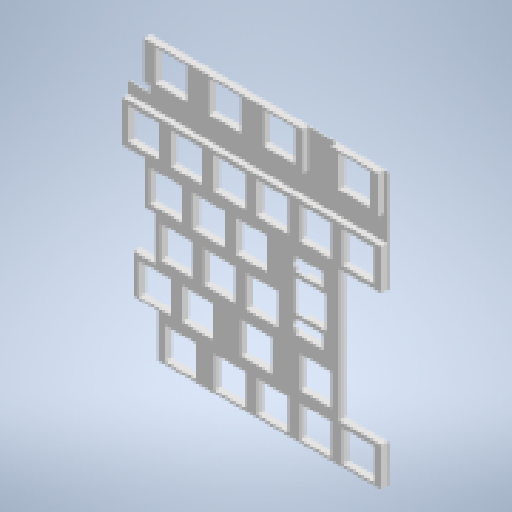
# Autodesk Inventor part: Right plate
Saved by Autodesk Inventor 2025 (Build 290162000, 162)
## iProperties
Created: 2024-08-01
Part Number: Right plate
Material: Generic
Document SubType Name: Modeling
Designer: adam
Density: 1 g/cm^3
Appearance: Default
Author: adam
Autodesk Inventor part; units mm, degrees
(part 1 of 2)
ref_plane "YZ Plane" through (0, 0, 0) normal (1, 0, 0) x (0, 1, 0)
ref_plane "XZ Plane" through (0, 0, 0) normal (0, 1, 0) x (-1, 0, 0)
ref_plane "XY Plane" through (0, 0, 0) normal (0, 0, 1) x (1, 0, 0)
sketch "Sketch1" plane through (0, 0, 0) normal (0, 0, 1) x (1, 0, 0)
  line L0 (210, -24.2525) -> (210, -19.005) construction
  line L1 (200.5, -24.2525) -> (210, -24.2525) construction
  line L2 (200.5, -29.5) -> (200.5, -24.2525) construction
  line L3 (200.5, -48.0525) -> (200.5, -29.5) construction
  line L4 (210.25, -48.0525) -> (200.5, -48.0525) construction
  line L5 (210.25, -67.1525) -> (210.25, -48.0525) construction
  line L6 (215, -67.1525) -> (210.25, -67.1525) construction
  line L7 (215, -86.2525) -> (215, -67.1525) construction
  line L8 (205.25, -86.2525) -> (215, -86.2525) construction
  line L9 (205.25, -103.805) -> (205.25, -86.2525) construction
  line L10 (216.3009, -103.805) -> (205.25, -103.805) construction
  line L11 (216.3009, -120.0025) -> (216.3009, -103.805) construction
  line L12 (210.1, -2) -> (210.1, -24.3525)
  line L13 (210.1, -24.3525) -> (200.6, -24.3525)
  line L14 (200.6, -24.3525) -> (200.6, -29.5)
  line L15 (200.6, -29.5) -> (200.6, -47.9525)
  line L16 (200.6, -47.9525) -> (210.35, -47.9525)
  line L17 (210.35, -47.9525) -> (210.35, -67.0525)
  line L18 (210.35, -67.0525) -> (215.1, -67.0525)
  line L19 (215.1, -67.0525) -> (215.1, -86.3525)
  line L20 (215.1, -86.3525) -> (205.35, -86.3525)
  line L21 (205.35, -86.3525) -> (205.35, -103.705)
  line L22 (205.35, -103.705) -> (216.4009, -103.705)
  line L23 (216.4009, -103.705) -> (216.4009, -123)
  line L24 (316, -2) -> (316, -123) projected
  line L25 (316, -2) -> (210.1, -2)
  line L26 (316, -123) -> (216.4009, -123)
  line L27 (316, -123) -> (0, -123) construction
  line L28 (316, -2) -> (316, -123) construction
  line L29 (0, -2) -> (316, -2) construction
  line L30 (0, -123) -> (0, -2) construction
  circle A0 centre (18.6, -119.6) radius 0.725 construction
  circle A1 centre (23, -114.9) radius 2.55 construction
  circle A2 centre (25.6, -120.65) radius 0.725 construction
  circle A3 centre (43.1, -119.6) radius 0.725 construction
  circle A4 centre (50.1, -120.65) radius 0.725 construction
  circle A5 centre (47.5, -114.9) radius 2.55 construction
  line L31 (67.3517, -120.975) -> (73.3517, -120.975) construction
  line L32 (67.3517, -105.975) -> (67.3517, -120.975) construction
  line L33 (73.3517, -105.975) -> (67.3517, -105.975) construction
  line L34 (73.3517, -120.975) -> (73.3517, -105.975) construction
  circle A6 centre (13.1, -100.5) radius 0.725 construction
  circle A7 centre (20.1, -101.55) radius 0.725 construction
  circle A8 centre (39.35, -100.5) radius 0.725 construction
  circle A9 centre (17.5, -95.8) radius 2.55 construction
  circle A10 centre (46.35, -101.55) radius 0.725 construction
  circle A11 centre (58.35, -100.5) radius 0.725 construction
  circle A12 centre (65.35, -101.55) radius 0.725 construction
  circle A13 centre (77.35, -100.5) radius 0.725 construction
  circle A14 centre (43.75, -95.8) radius 2.55 construction
  circle A15 centre (62.75, -95.8) radius 2.55 construction
  circle A16 centre (81.75, -95.8) radius 2.55 construction
  circle A17 centre (132.4518, -119.675) radius 0.725 construction
  circle A18 centre (139.4518, -120.725) radius 0.725 construction
  circle A19 centre (136.8518, -114.975) radius 2.55 construction
  circle A20 centre (84.35, -101.55) radius 0.725 construction
  circle A21 centre (96.35, -100.5) radius 0.725 construction
  circle A22 centre (103.35, -101.55) radius 0.725 construction
  circle A23 centre (115.35, -100.5) radius 0.725 construction
  circle A24 centre (100.75, -95.8) radius 2.55 construction
  circle A25 centre (119.75, -95.8) radius 2.55 construction
  circle A26 centre (122.35, -101.55) radius 0.725 construction
  circle A27 centre (134.35, -100.5) radius 0.725 construction
  circle A28 centre (141.35, -101.55) radius 0.725 construction
  circle A29 centre (153.35, -100.5) radius 0.725 construction
  circle A30 centre (138.75, -95.8) radius 2.55 construction
  circle A31 centre (157.75, -95.8) radius 2.55 construction
  circle A32 centre (15.6, -82.45) radius 0.725 construction
  circle A33 centre (8.6, -81.4) radius 0.725 construction
  circle A34 centre (37.1, -82.45) radius 0.725 construction
  circle A35 centre (30.1, -81.4) radius 0.725 construction
  circle A36 centre (56.1, -82.45) radius 0.725 construction
  circle A37 centre (49.1, -81.4) radius 0.725 construction
  circle A38 centre (75.1, -82.45) radius 0.725 construction
  circle A39 centre (68.1, -81.4) radius 0.725 construction
  circle A40 centre (13, -76.7) radius 2.55 construction
  circle A41 centre (34.5, -76.7) radius 2.55 construction
  circle A42 centre (53.5, -76.7) radius 2.55 construction
  circle A43 centre (72.5, -76.7) radius 2.55 construction
  circle A44 centre (94.1, -82.45) radius 0.725 construction
  circle A45 centre (87.1, -81.4) radius 0.725 construction
  circle A46 centre (113.1, -82.45) radius 0.725 construction
  circle A47 centre (106.1, -81.4) radius 0.725 construction
  circle A48 centre (132.1, -82.45) radius 0.725 construction
  circle A49 centre (125.1, -81.4) radius 0.725 construction
  circle A50 centre (151.1, -82.45) radius 0.725 construction
  circle A51 centre (144.1, -81.4) radius 0.725 construction
  circle A52 centre (91.5, -76.7) radius 2.55 construction
  circle A53 centre (110.5, -76.7) radius 2.55 construction
  circle A54 centre (129.5, -76.7) radius 2.55 construction
  circle A55 centre (148.5, -76.7) radius 2.55 construction
  circle A56 centre (221.85, -119.6) radius 0.725 construction
  circle A57 centre (228.85, -120.65) radius 0.725 construction
  circle A58 centre (226.25, -114.9) radius 2.55 construction
  line L35 (200.3518, -120.975) -> (206.3518, -120.975) construction
  line L36 (200.3518, -105.975) -> (200.3518, -120.975) construction
  line L37 (206.3518, -105.975) -> (200.3518, -105.975) construction
  line L38 (206.3518, -120.975) -> (206.3518, -105.975) construction
  circle A59 centre (160.35, -101.55) radius 0.725 construction
  circle A60 centre (172.35, -100.5) radius 0.725 construction
  circle A61 centre (179.35, -101.55) radius 0.725 construction
  circle A62 centre (191.35, -100.5) radius 0.725 construction
  circle A63 centre (198.35, -101.55) radius 0.725 construction
  circle A64 centre (176.75, -95.8) radius 2.55 construction
  circle A65 centre (195.75, -95.8) radius 2.55 construction
  circle A66 centre (210.35, -100.5) radius 0.725 construction
  circle A67 centre (217.35, -101.55) radius 0.725 construction
  circle A68 centre (229.35, -100.5) radius 0.725 construction
  circle A69 centre (236.35, -101.55) radius 0.725 construction
  circle A70 centre (214.75, -95.8) radius 2.55 construction
  circle A71 centre (233.75, -95.8) radius 2.55 construction
  circle A72 centre (243.85, -119.6) radius 0.725 construction
  circle A73 centre (250.85, -120.65) radius 0.725 construction
  circle A74 centre (248.25, -114.9) radius 2.55 construction
  circle A75 centre (262.85, -119.6) radius 0.725 construction
  circle A76 centre (269.85, -120.65) radius 0.725 construction
  circle A77 centre (267.25, -114.9) radius 2.55 construction
  circle A78 centre (281.85, -119.6) radius 0.725 construction
  circle A79 centre (288.85, -120.65) radius 0.725 construction
  circle A80 centre (286.25, -114.9) radius 2.55 construction
  circle A81 centre (300.85, -119.6) radius 0.725 construction
  circle A82 centre (307.85, -120.65) radius 0.725 construction
  circle A83 centre (305.25, -114.9) radius 2.55 construction
  circle A84 centre (255.6, -100.5) radius 0.725 construction
  circle A85 centre (262.6, -101.55) radius 0.725 construction
  circle A86 centre (260, -95.8) radius 2.55 construction
  circle A87 centre (281.85, -100.5) radius 0.725 construction
  circle A88 centre (288.85, -101.55) radius 0.725 construction
  circle A89 centre (314, -102.5) radius 0.5 construction
  circle A90 centre (286.25, -95.8) radius 2.55 construction
  circle A91 centre (314, -99.96) radius 0.5 construction
  circle A92 centre (314, -97.42) radius 0.5 construction
  circle A93 centre (314, -94.88) radius 0.5 construction
  circle A94 centre (170.1, -82.45) radius 0.725 construction
  circle A95 centre (163.1, -81.4) radius 0.725 construction
  circle A96 centre (189.1, -82.45) radius 0.725 construction
  circle A97 centre (182.1, -81.4) radius 0.725 construction
  circle A98 centre (208.1, -82.45) radius 0.725 construction
  circle A99 centre (201.1, -81.4) radius 0.725 construction
  circle A100 centre (227.1, -82.45) radius 0.725 construction
  circle A101 centre (220.1, -81.4) radius 0.725 construction
  circle A102 centre (167.5, -76.7) radius 2.55 construction
  circle A103 centre (186.5, -76.7) radius 2.55 construction
  circle A104 centre (205.5, -76.7) radius 2.55 construction
  circle A105 centre (224.5, -76.7) radius 2.55 construction
  circle A106 centre (246.1, -82.45) radius 0.725 construction
  circle A107 centre (239.1, -81.4) radius 0.725 construction
  circle A108 centre (265.1, -82.45) radius 0.725 construction
  circle A109 centre (258.1, -81.4) radius 0.725 construction
  circle A110 centre (314, -92.34) radius 0.5 construction
  circle A111 centre (314, -89.8) radius 0.5 construction
  line L39 (275, -82.25) -> (290, -82.25) construction
  line L40 (275, -76.25) -> (275, -82.25) construction
  line L41 (290, -76.25) -> (275, -76.25) construction
  line L42 (290, -82.25) -> (290, -76.25) construction
  circle A112 centre (243.5, -76.7) radius 2.55 construction
  circle A113 centre (262.5, -76.7) radius 2.55 construction
  circle A114 centre (288.675, -71.675) radius 0.725 construction
  circle A115 centre (283.975, -67.275) radius 2.55 construction
  circle A116 centre (289.725, -64.675) radius 0.725 construction
  circle A117 centre (22.6, -63.35) radius 0.725 construction
  circle A118 centre (15.6, -62.3) radius 0.725 construction
  circle A119 centre (20, -57.6) radius 2.55 construction
  line L43 (5, -63.6) -> (11, -63.6) construction
  line L44 (5, -48.6) -> (5, -63.6) construction
  line L45 (11, -48.6) -> (5, -48.6) construction
  line L46 (11, -63.6) -> (11, -48.6) construction
  line L47 (29, -63.6) -> (35, -63.6) construction
  line L48 (29, -48.6) -> (29, -63.6) construction
  line L49 (35, -48.6) -> (29, -48.6) construction
  line L50 (35, -63.6) -> (35, -48.6) construction
  circle A120 centre (51.35, -63.35) radius 0.725 construction
  circle A121 centre (44.35, -62.3) radius 0.725 construction
  circle A122 centre (48.75, -57.6) radius 2.55 construction
  circle A123 centre (70.35, -63.35) radius 0.725 construction
  circle A124 centre (63.35, -62.3) radius 0.725 construction
  circle A125 centre (82.35, -62.3) radius 0.725 construction
  circle A126 centre (67.75, -57.6) radius 2.55 construction
  circle A127 centre (10.6, -43.2) radius 0.725 construction
  circle A128 centre (17.6, -44.25) radius 0.725 construction
  circle A129 centre (34.6, -43.2) radius 0.725 construction
  circle A130 centre (41.6, -44.25) radius 0.725 construction
  circle A131 centre (15, -38.5) radius 2.55 construction
  circle A132 centre (39, -38.5) radius 2.55 construction
  circle A133 centre (53.6, -43.2) radius 0.725 construction
  circle A134 centre (60.6, -44.25) radius 0.725 construction
  circle A135 centre (72.6, -43.2) radius 0.725 construction
  circle A136 centre (79.6, -44.25) radius 0.725 construction
  circle A137 centre (58, -38.5) radius 2.55 construction
  circle A138 centre (77, -38.5) radius 2.55 construction
  circle A139 centre (89.35, -63.35) radius 0.725 construction
  circle A140 centre (101.35, -62.3) radius 0.725 construction
  circle A141 centre (86.75, -57.6) radius 2.55 construction
  circle A142 centre (108.35, -63.35) radius 0.725 construction
  circle A143 centre (120.35, -62.3) radius 0.725 construction
  circle A144 centre (105.75, -57.6) radius 2.55 construction
  circle A145 centre (127.35, -63.35) radius 0.725 construction
  circle A146 centre (139.35, -62.3) radius 0.725 construction
  circle A147 centre (124.75, -57.6) radius 2.55 construction
  circle A148 centre (146.35, -63.35) radius 0.725 construction
  circle A149 centre (158.35, -62.3) radius 0.725 construction
  circle A150 centre (143.75, -57.6) radius 2.55 construction
  circle A151 centre (91.6, -43.2) radius 0.725 construction
  circle A152 centre (98.6, -44.25) radius 0.725 construction
  circle A153 centre (110.6, -43.2) radius 0.725 construction
  circle A154 centre (117.6, -44.25) radius 0.725 construction
  circle A155 centre (96, -38.5) radius 2.55 construction
  circle A156 centre (115, -38.5) radius 2.55 construction
  circle A157 centre (129.6, -43.2) radius 0.725 construction
  circle A158 centre (136.6, -44.25) radius 0.725 construction
  circle A159 centre (148.6, -43.2) radius 0.725 construction
  circle A160 centre (155.6, -44.25) radius 0.725 construction
  circle A161 centre (134, -38.5) radius 2.55 construction
  circle A162 centre (153, -38.5) radius 2.55 construction
  circle A163 centre (8.1, -14.7) radius 0.725 construction
  circle A164 centre (15.1, -15.75) radius 0.725 construction
  circle A165 centre (41.1, -14.7) radius 0.725 construction
  circle A166 centre (12.5, -10) radius 2.55 construction
  circle A167 centre (48.1, -15.75) radius 0.725 construction
  circle A168 centre (65.1, -14.7) radius 0.725 construction
  circle A169 centre (72.1, -15.75) radius 0.725 construction
  circle A170 centre (45.5, -10) radius 2.55 construction
  circle A171 centre (69.5, -10) radius 2.55 construction
  circle A172 centre (123.5, -26.25) radius 0.425 construction
  circle A173 centre (126, -26.25) radius 0.425 construction
  circle A174 centre (128.5, -26.25) radius 0.425 construction
  circle A175 centre (131, -26.25) radius 0.425 construction
  circle A176 centre (133.5, -26.25) radius 0.425 construction
  circle A177 centre (136, -26.25) radius 0.425 construction
  circle A178 centre (138.5, -26.25) radius 0.425 construction
  circle A179 centre (122.25, -23.75) radius 0.425 construction
  circle A180 centre (124.75, -23.75) radius 0.425 construction
  circle A181 centre (127.25, -23.75) radius 0.425 construction
  circle A182 centre (129.75, -23.75) radius 0.425 construction
  circle A183 centre (132.25, -23.75) radius 0.425 construction
  circle A184 centre (134.75, -23.75) radius 0.425 construction
  circle A185 centre (137.25, -23.75) radius 0.425 construction
  circle A186 centre (139.75, -23.75) radius 0.425 construction
  circle A187 centre (141, -26.25) radius 0.425 construction
  circle A188 centre (143.5, -26.25) radius 0.425 construction
  circle A189 centre (146, -26.25) radius 0.425 construction
  circle A190 centre (148.5, -26.25) radius 0.425 construction
  circle A191 centre (151, -26.25) radius 0.425 construction
  circle A192 centre (153.5, -26.25) radius 0.425 construction
  circle A193 centre (156, -26.25) radius 0.425 construction
  circle A194 centre (158.5, -26.25) radius 0.425 construction
  circle A195 centre (142.25, -23.75) radius 0.425 construction
  circle A196 centre (144.75, -23.75) radius 0.425 construction
  circle A197 centre (147.25, -23.75) radius 0.425 construction
  circle A198 centre (149.75, -23.75) radius 0.425 construction
  circle A199 centre (152.25, -23.75) radius 0.425 construction
  circle A200 centre (154.75, -23.75) radius 0.425 construction
  circle A201 centre (157.25, -23.75) radius 0.425 construction
  circle A202 centre (89.1, -14.7) radius 0.725 construction
  circle A203 centre (96.1, -15.75) radius 0.725 construction
  circle A204 centre (113.1, -14.7) radius 0.725 construction
  circle A205 centre (120.1, -15.75) radius 0.725 construction
  circle A206 centre (93.5, -10) radius 2.55 construction
  circle A207 centre (117.5, -10) radius 2.55 construction
  circle A208 centre (137.1, -14.7) radius 0.725 construction
  circle A209 centre (144.1, -15.75) radius 0.725 construction
  circle A210 centre (141.5, -10) radius 2.55 construction
  circle A211 centre (165.35, -63.35) radius 0.725 construction
  circle A212 centre (177.35, -62.3) radius 0.725 construction
  circle A213 centre (162.75, -57.6) radius 2.55 construction
  circle A214 centre (184.35, -63.35) radius 0.725 construction
  circle A215 centre (196.35, -62.3) radius 0.725 construction
  circle A216 centre (181.75, -57.6) radius 2.55 construction
  circle A217 centre (203.35, -63.35) radius 0.725 construction
  circle A218 centre (215.35, -62.3) radius 0.725 construction
  circle A219 centre (200.75, -57.6) radius 2.55 construction
  circle A220 centre (222.35, -63.35) radius 0.725 construction
  circle A221 centre (234.35, -62.45) radius 0.725 construction
  circle A222 centre (219.75, -57.6) radius 2.55 construction
  circle A223 centre (167.6, -43.2) radius 0.725 construction
  circle A224 centre (174.6, -44.25) radius 0.725 construction
  circle A225 centre (186.6, -43.2) radius 0.725 construction
  circle A226 centre (193.6, -44.25) radius 0.725 construction
  circle A227 centre (172, -38.5) radius 2.55 construction
  circle A228 centre (191, -38.5) radius 2.55 construction
  circle A229 centre (205.6, -43.2) radius 0.725 construction
  circle A230 centre (212.6, -44.25) radius 0.725 construction
  circle A231 centre (224.6, -43.2) radius 0.725 construction
  circle A232 centre (231.6, -44.25) radius 0.725 construction
  circle A233 centre (210, -38.5) radius 2.55 construction
  circle A234 centre (229, -38.5) radius 2.55 construction
  circle A235 centre (241.35, -63.5) radius 0.725 construction
  circle A236 centre (253.35, -62.4466) radius 0.725 construction
  circle A237 centre (238.75, -57.75) radius 2.55 construction
  circle A238 centre (260.35, -63.4966) radius 0.725 construction
  circle A239 centre (257.75, -57.7466) radius 2.55 construction
  line L51 (275, -58.25) -> (290, -58.25) construction
  line L52 (275, -52.25) -> (275, -58.25) construction
  line L53 (290, -52.25) -> (275, -52.25) construction
  line L54 (290, -58.25) -> (290, -52.25) construction
  circle A240 centre (243.6, -43.2) radius 0.725 construction
  circle A241 centre (250.6, -44.25) radius 0.725 construction
  circle A242 centre (262.6, -43.2) radius 0.725 construction
  circle A243 centre (269.6, -44.25) radius 0.725 construction
  circle A244 centre (248, -38.5) radius 2.55 construction
  circle A245 centre (267, -38.5) radius 2.55 construction
  circle A246 centre (281.6, -43.2) radius 0.725 construction
  circle A247 centre (288.6, -44.25) radius 0.725 construction
  circle A248 centre (300.6, -43.2) radius 0.725 construction
  circle A249 centre (307.6, -44.25) radius 0.725 construction
  circle A250 centre (286, -38.5) radius 2.55 construction
  circle A251 centre (305, -38.5) radius 2.55 construction
  circle A252 centre (161, -26.25) radius 0.425 construction
  circle A253 centre (159.75, -23.75) radius 0.425 construction
  circle A254 centre (219, -34) radius 1.6 construction
  circle A255 centre (169.6, -14.7) radius 0.725 construction
  circle A256 centre (176.6, -15.75) radius 0.725 construction
  circle A257 centre (193.6, -14.7) radius 0.725 construction
  circle A258 centre (174, -10) radius 2.55 construction
  circle A259 centre (198, -10) radius 2.55 construction
  circle A260 centre (200.6, -15.75) radius 0.725 construction
  circle A261 centre (217.6, -14.7) radius 0.725 construction
  circle A262 centre (224.6, -15.75) radius 0.725 construction
  circle A263 centre (222, -10) radius 2.55 construction
  circle A264 centre (241.6, -14.7) radius 0.725 construction
  circle A265 centre (248.6, -15.75) radius 0.725 construction
  circle A266 centre (265.6, -14.7) radius 0.725 construction
  circle A267 centre (272.6, -15.75) radius 0.725 construction
  circle A268 centre (246, -10) radius 2.55 construction
  circle A269 centre (270, -10) radius 2.55 construction
  circle A270 centre (299.1, -14.7) radius 0.725 construction
  circle A271 centre (306.1, -15.75) radius 0.725 construction
  circle A272 centre (303.5, -10) radius 2.55 construction
  line L55 (214.9975, -2.9975) -> (229.0025, -2.9975)
  line L56 (229.0025, -2.9975) -> (229.0025, -17.0025)
  line L57 (229.0025, -17.0025) -> (214.9975, -17.0025)
  line L58 (214.9975, -17.0025) -> (214.9975, -2.9975)
  line L59 (214.9975, -2.9975) -> (229.0025, -17.0025) construction
  line L60 (229.0025, -2.9975) -> (214.9975, -17.0025) construction
  line L61 (238.9975, -2.9975) -> (253.0025, -2.9975)
  line L62 (253.0025, -2.9975) -> (253.0025, -17.0025)
  line L63 (253.0025, -17.0025) -> (238.9975, -17.0025)
  line L64 (238.9975, -17.0025) -> (238.9975, -2.9975)
  line L65 (238.9975, -2.9975) -> (253.0025, -17.0025) construction
  line L66 (253.0025, -2.9975) -> (238.9975, -17.0025) construction
  line L67 (262.9975, -2.9975) -> (277.0025, -2.9975)
  line L68 (277.0025, -2.9975) -> (277.0025, -17.0025)
  line L69 (277.0025, -17.0025) -> (262.9975, -17.0025)
  line L70 (262.9975, -17.0025) -> (262.9975, -2.9975)
  line L71 (262.9975, -2.9975) -> (277.0025, -17.0025) construction
  line L72 (277.0025, -2.9975) -> (262.9975, -17.0025) construction
  line L73 (296.4975, -2.9975) -> (310.5025, -2.9975)
  line L74 (310.5025, -2.9975) -> (310.5025, -17.0025)
  line L75 (310.5025, -17.0025) -> (296.4975, -17.0025)
  line L76 (296.4975, -17.0025) -> (296.4975, -2.9975)
  line L77 (296.4975, -2.9975) -> (310.5025, -17.0025) construction
  line L78 (310.5025, -2.9975) -> (296.4975, -17.0025) construction
  line L79 (202.9975, -31.4975) -> (217.0025, -31.4975)
  line L80 (217.0025, -31.4975) -> (217.0025, -45.5025)
  line L81 (217.0025, -45.5025) -> (202.9975, -45.5025)
  line L82 (202.9975, -45.5025) -> (202.9975, -31.4975)
  line L83 (202.9975, -31.4975) -> (217.0025, -45.5025) construction
  line L84 (217.0025, -31.4975) -> (202.9975, -45.5025) construction
  line L85 (221.9975, -31.4975) -> (236.0025, -31.4975)
  line L86 (236.0025, -31.4975) -> (236.0025, -45.5025)
  line L87 (236.0025, -45.5025) -> (221.9975, -45.5025)
  line L88 (221.9975, -45.5025) -> (221.9975, -31.4975)
  line L89 (221.9975, -31.4975) -> (236.0025, -45.5025) construction
  line L90 (236.0025, -31.4975) -> (221.9975, -45.5025) construction
  line L91 (240.9975, -31.4975) -> (255.0025, -31.4975)
  line L92 (255.0025, -31.4975) -> (255.0025, -45.5025)
  line L93 (255.0025, -45.5025) -> (240.9975, -45.5025)
  line L94 (240.9975, -45.5025) -> (240.9975, -31.4975)
  line L95 (240.9975, -31.4975) -> (255.0025, -45.5025) construction
  line L96 (255.0025, -31.4975) -> (240.9975, -45.5025) construction
  line L97 (259.9975, -31.4975) -> (274.0025, -31.4975)
  line L98 (274.0025, -31.4975) -> (274.0025, -45.5025)
  line L99 (274.0025, -45.5025) -> (259.9975, -45.5025)
  line L100 (259.9975, -45.5025) -> (259.9975, -31.4975)
  line L101 (259.9975, -31.4975) -> (274.0025, -45.5025) construction
  line L102 (274.0025, -31.4975) -> (259.9975, -45.5025) construction
  line L103 (278.9975, -31.4975) -> (293.0025, -31.4975)
  line L104 (293.0025, -31.4975) -> (293.0025, -45.5025)
  line L105 (293.0025, -45.5025) -> (278.9975, -45.5025)
  line L106 (278.9975, -45.5025) -> (278.9975, -31.4975)
  line L107 (278.9975, -31.4975) -> (293.0025, -45.5025) construction
  line L108 (293.0025, -31.4975) -> (278.9975, -45.5025) construction
  line L109 (297.9975, -31.4975) -> (312.0025, -31.4975)
  line L110 (312.0025, -31.4975) -> (312.0025, -45.5025)
  line L111 (312.0025, -45.5025) -> (297.9975, -45.5025)
  line L112 (297.9975, -45.5025) -> (297.9975, -31.4975)
  line L113 (297.9975, -31.4975) -> (312.0025, -45.5025) construction
  line L114 (312.0025, -31.4975) -> (297.9975, -45.5025) construction
  line L115 (212.7475, -50.5975) -> (226.7525, -50.5975)
  line L116 (226.7525, -50.5975) -> (226.7525, -64.6025)
  line L117 (226.7525, -64.6025) -> (212.7475, -64.6025)
  line L118 (212.7475, -64.6025) -> (212.7475, -50.5975)
  line L119 (212.7475, -50.5975) -> (226.7525, -64.6025) construction
  line L120 (226.7525, -50.5975) -> (212.7475, -64.6025) construction
  line L121 (231.7475, -50.7475) -> (245.7525, -50.7475)
  line L122 (245.7525, -50.7475) -> (245.7525, -64.7525)
  line L123 (245.7525, -64.7525) -> (231.7475, -64.7525)
  line L124 (231.7475, -64.7525) -> (231.7475, -50.7475)
  line L125 (231.7475, -50.7475) -> (245.7525, -64.7525) construction
  line L126 (245.7525, -50.7475) -> (231.7475, -64.7525) construction
  line L127 (250.7475, -50.7441) -> (264.7525, -50.7441)
  line L128 (264.7525, -50.7441) -> (264.7525, -64.7491)
  line L129 (264.7525, -64.7491) -> (250.7475, -64.7491)
  line L130 (250.7475, -64.7491) -> (250.7475, -50.7441)
  line L131 (250.7475, -50.7441) -> (264.7525, -64.7491) construction
  line L132 (264.7525, -50.7441) -> (250.7475, -64.7491) construction
  line L133 (217.4975, -69.6975) -> (231.5025, -69.6975)
  line L134 (231.5025, -69.6975) -> (231.5025, -83.7025)
  line L135 (231.5025, -83.7025) -> (217.4975, -83.7025)
  line L136 (217.4975, -83.7025) -> (217.4975, -69.6975)
  line L137 (217.4975, -69.6975) -> (231.5025, -83.7025) construction
  line L138 (231.5025, -69.6975) -> (217.4975, -83.7025) construction
  line L139 (236.4975, -69.6975) -> (250.5025, -69.6975)
  line L140 (250.5025, -69.6975) -> (250.5025, -83.7025)
  line L141 (250.5025, -83.7025) -> (236.4975, -83.7025)
  line L142 (236.4975, -83.7025) -> (236.4975, -69.6975)
  line L143 (236.4975, -69.6975) -> (250.5025, -83.7025) construction
  line L144 (250.5025, -69.6975) -> (236.4975, -83.7025) construction
  line L145 (255.4975, -69.6975) -> (269.5025, -69.6975)
  line L146 (269.5025, -69.6975) -> (269.5025, -83.7025)
  line L147 (269.5025, -83.7025) -> (255.4975, -83.7025)
  line L148 (255.4975, -83.7025) -> (255.4975, -69.6975)
  line L149 (255.4975, -69.6975) -> (269.5025, -83.7025) construction
  line L150 (269.5025, -69.6975) -> (255.4975, -83.7025) construction
  line L151 (207.7475, -88.7975) -> (221.7525, -88.7975)
  line L152 (221.7525, -88.7975) -> (221.7525, -102.8025)
  line L153 (221.7525, -102.8025) -> (207.7475, -102.8025)
  line L154 (207.7475, -102.8025) -> (207.7475, -88.7975)
  line L155 (207.7475, -88.7975) -> (221.7525, -102.8025) construction
  line L156 (221.7525, -88.7975) -> (207.7475, -102.8025) construction
  line L157 (226.7475, -88.7975) -> (240.7525, -88.7975)
  line L158 (240.7525, -88.7975) -> (240.7525, -102.8025)
  line L159 (240.7525, -102.8025) -> (226.7475, -102.8025)
  line L160 (226.7475, -102.8025) -> (226.7475, -88.7975)
  line L161 (226.7475, -88.7975) -> (240.7525, -102.8025) construction
  line L162 (240.7525, -88.7975) -> (226.7475, -102.8025) construction
  line L163 (252.9975, -88.7975) -> (267.0025, -88.7975)
  line L164 (267.0025, -88.7975) -> (267.0025, -102.8025)
  line L165 (267.0025, -102.8025) -> (252.9975, -102.8025)
  line L166 (252.9975, -102.8025) -> (252.9975, -88.7975)
  line L167 (252.9975, -88.7975) -> (267.0025, -102.8025) construction
  line L168 (267.0025, -88.7975) -> (252.9975, -102.8025) construction
  line L169 (279.2475, -88.7975) -> (293.2525, -88.7975)
  line L170 (293.2525, -88.7975) -> (293.2525, -102.8025)
  line L171 (293.2525, -102.8025) -> (279.2475, -102.8025)
  line L172 (279.2475, -102.8025) -> (279.2475, -88.7975)
  line L173 (279.2475, -88.7975) -> (293.2525, -102.8025) construction
  line L174 (293.2525, -88.7975) -> (279.2475, -102.8025) construction
  line L175 (219.2475, -107.8975) -> (233.2525, -107.8975)
  line L176 (233.2525, -107.8975) -> (233.2525, -121.9025)
  line L177 (233.2525, -121.9025) -> (219.2475, -121.9025)
  line L178 (219.2475, -121.9025) -> (219.2475, -107.8975)
  line L179 (219.2475, -107.8975) -> (233.2525, -121.9025) construction
  line L180 (233.2525, -107.8975) -> (219.2475, -121.9025) construction
  line L181 (241.2475, -107.8975) -> (255.2525, -107.8975)
  line L182 (255.2525, -107.8975) -> (255.2525, -121.9025)
  line L183 (255.2525, -121.9025) -> (241.2475, -121.9025)
  line L184 (241.2475, -121.9025) -> (241.2475, -107.8975)
  line L185 (241.2475, -107.8975) -> (255.2525, -121.9025) construction
  line L186 (255.2525, -107.8975) -> (241.2475, -121.9025) construction
  line L187 (260.2475, -107.8975) -> (274.2525, -107.8975)
  line L188 (274.2525, -107.8975) -> (274.2525, -121.9025)
  line L189 (274.2525, -121.9025) -> (260.2475, -121.9025)
  line L190 (260.2475, -121.9025) -> (260.2475, -107.8975)
  line L191 (260.2475, -107.8975) -> (274.2525, -121.9025) construction
  line L192 (274.2525, -107.8975) -> (260.2475, -121.9025) construction
  line L193 (279.2475, -107.8975) -> (293.2525, -107.8975)
  line L194 (293.2525, -107.8975) -> (293.2525, -121.9025)
  line L195 (293.2525, -121.9025) -> (279.2475, -121.9025)
  line L196 (279.2475, -121.9025) -> (279.2475, -107.8975)
  line L197 (279.2475, -107.8975) -> (293.2525, -121.9025) construction
  line L198 (293.2525, -107.8975) -> (279.2475, -121.9025) construction
  line L199 (298.2475, -107.8975) -> (312.2525, -107.8975)
  line L200 (312.2525, -107.8975) -> (312.2525, -121.9025)
  line L201 (312.2525, -121.9025) -> (298.2475, -121.9025)
  line L202 (298.2475, -121.9025) -> (298.2475, -107.8975)
  line L203 (298.2475, -107.8975) -> (312.2525, -121.9025) construction
  line L204 (312.2525, -107.8975) -> (298.2475, -121.9025) construction
  line L205 (276.9725, -60.2725) -> (290.9775, -60.2725)
  line L206 (290.9775, -60.2725) -> (290.9775, -74.2775)
  line L207 (290.9775, -74.2775) -> (276.9725, -74.2775)
  line L208 (276.9725, -74.2775) -> (276.9725, -60.2725)
  line L209 (276.9725, -60.2725) -> (290.9775, -74.2775) construction
  line L210 (290.9775, -60.2725) -> (276.9725, -74.2775) construction
  line L211 (277.2225, -58.375) -> (289.7225, -58.375)
  line L212 (289.7225, -58.375) -> (289.7225, -52.375)
  line L213 (289.7225, -52.375) -> (277.2225, -52.375)
  line L214 (277.2225, -52.375) -> (277.2225, -58.375)
  line L215 (277.2225, -76.175) -> (289.7225, -76.175)
  line L216 (289.7225, -76.175) -> (289.7225, -82.175)
  line L217 (289.7225, -82.175) -> (277.2225, -82.175)
  line L218 (277.2225, -82.175) -> (277.2225, -76.175)
  line L219 (277.2225, -55.375) -> (289.7225, -55.375) construction
  line L220 (277.2225, -79.175) -> (289.7225, -79.175) construction
  line L221 (316, -2) -> (316, -47.5025)
  line L222 (316, -47.5025) -> (296.7525, -47.5025)
  line L223 (296.7525, -47.5025) -> (296.7525, -105.8975)
  line L224 (296.7525, -105.8975) -> (316, -105.8975)
  line L225 (316, -105.8975) -> (316, -123)
  point P0 (0, 0)
  dimension "d0" = 0.1
  dimension "d1" = 0.1
  dimension "d2" = 14.005
  dimension "d3" = 14.005
  dimension "d4" = 14.005
  dimension "d5" = 14.005
  dimension "d6" = 14.005
  dimension "d7" = 14.005
  dimension "d8" = 14.005
  dimension "d9" = 14.005
  dimension "d10" = 14.005
  dimension "d11" = 14.005
  dimension "d12" = 14.005
  dimension "d13" = 14.005
  dimension "d14" = 14.005
  dimension "d15" = 14.005
  dimension "d16" = 14.005
  dimension "d17" = 14.005
  dimension "d18" = 14.005
  dimension "d19" = 14.005
  dimension "d20" = 14.005
  dimension "d21" = 14.005
  dimension "d22" = 14.005
  dimension "d23" = 14.005
  dimension "d24" = 14.005
  dimension "d25" = 14.005
  dimension "d26" = 14.005
  dimension "d27" = 14.005
  dimension "d30" = 14.005
  dimension "d31" = 14.005
  dimension "d32" = 14.005
  dimension "d33" = 14.005
  dimension "d34" = 14.005
  dimension "d35" = 14.005
  dimension "d36" = 14.005
  dimension "d37" = 14.005
  dimension "d38" = 14.005
  dimension "d39" = 14.005
  dimension "d40" = 14.005
  dimension "d41" = 14.005
  dimension "d42" = 14.005
  dimension "d43" = 14.005
  dimension "d44" = 14.005
  dimension "d45" = 14.005
  dimension "d46" = 14.005
  dimension "d47" = 14.005
  dimension "d48" = 14.005
  dimension "d49" = 14.005
  dimension "d50" = 14.005
  dimension "d51" = 14.005
  dimension "d52" = 14.005
  dimension "d53" = 14.005
  dimension "d55" = 14.005
  dimension "d56" = 14.005
  dimension "d57" = 11.9
  dimension "d58" = 11.9
  dimension "d59" = 6
  dimension "d60" = 12.5
  dimension "d79" = 2
  dimension "d80" = 2
  dimension "d81" = 3.5
  dimension "d93" = 0.25
  constraints: 372 end point, 56 midpoint, 56 parallel, 31 horizontal, 30 perpendicular, 4 point on line, 2 collinear, 11 other
  measures "d0" distance between parallel lines of L0 L12
  measures "d1" distance between parallel lines of L23 L11
  measures "d2" distance of L56.end L57.end
  measures "d3" distance of L55.end L56.end
  measures "d4" distance of L62.end L63.end
  measures "d5" distance of L61.end L62.end
  measures "d6" distance of L68.end L69.end
  measures "d7" distance of L67.end L68.end
  measures "d8" distance of L74.end L75.end
  measures "d9" distance of L73.end L74.end
  measures "d10" distance of L80.end L81.end
  measures "d11" distance of L79.end L80.end
  measures "d12" distance of L86.end L87.end
  measures "d13" distance of L85.end L86.end
  measures "d14" distance of L92.end L93.end
  measures "d15" distance of L91.end L92.end
  measures "d16" distance of L98.end L99.end
  measures "d17" distance of L97.end L98.end
  measures "d18" distance of L104.end L105.end
  measures "d19" distance of L103.end L104.end
  measures "d20" distance of L110.end L111.end
  measures "d21" distance of L109.end L110.end
  measures "d22" distance of L116.end L117.end
  measures "d23" distance of L115.end L116.end
  measures "d24" distance of L122.end L123.end
  measures "d25" distance of L121.end L122.end
  measures "d26" distance of L128.end L129.end
  measures "d27" distance of L127.end L128.end
  measures "d30" distance of L134.end L135.end
  measures "d31" distance of L133.end L134.end
  measures "d32" distance of L140.end L141.end
  measures "d33" distance of L139.end L140.end
  measures "d34" distance of L146.end L147.end
  measures "d35" distance of L145.end L146.end
  measures "d36" distance of L152.end L153.end
  measures "d37" distance of L151.end L152.end
  measures "d38" distance of L158.end L159.end
  measures "d39" distance of L157.end L158.end
  measures "d40" distance of L164.end L165.end
  measures "d41" distance of L163.end L164.end
  measures "d42" distance of L170.end L171.end
  measures "d43" distance of L169.end L170.end
  measures "d44" distance of L176.end L177.end
  measures "d45" distance of L175.end L176.end
  measures "d46" distance of L182.end L183.end
  measures "d47" distance of L181.end L182.end
  measures "d48" distance of L188.end L189.end
  measures "d49" distance of L187.end L188.end
  measures "d50" distance of L194.end L195.end
  measures "d51" distance of L193.end L194.end
  measures "d52" distance of L200.end L201.end
  measures "d53" distance of L199.end L200.end
  measures "d55" distance of L206.end L207.end
  measures "d56" distance of L205.end L206.end
  measures "d57" distance from line of L220 A115.centre
  measures "d58" distance from line of L219 A115.centre
  measures "d59" distance of L217.end L215.start
  measures "d60" distance between parallel lines of L212 L214
  measures "d79" distance between parallel lines of L224 L199
  measures "d80" distance between parallel lines of L111 L222
  measures "d81" distance between parallel lines of L223 L170
  measures "d93" distance between parallel lines of L208 L214
extrude "Extrusion1" add sketch "Sketch1" along normal blind 0.5 contours L25 L24 L222 L223 L224 L26 L23 L22 L21 L20 L19 L18 L17 L16 L15 L14 L13 L12
sketch "Sketch2" plane through (0, 0, 0.5) normal (0, 0, 1) x (1, 0, 0)
  line L0 (210.1, -2) -> (210.1, -24.3525) projected
  line L1 (210.1, -19.0025) -> (280.5025, -19.0025)
  line L2 (280.5025, -19.0025) -> (280.5025, -2) construction
  line L3 (280.5025, -2) -> (210.1, -2)
  line L4 (210.1, -2) -> (210.1, -19.0025)
  line L5 (316, -2) -> (210.1, -2) projected
  line L6 (292.9975, -2) -> (292.9975, -19.0025)
  line L7 (292.9975, -19.0025) -> (314.0025, -19.0025)
  line L8 (314.0025, -19.0025) -> (314.0025, -2)
  line L9 (314.0025, -2) -> (292.9975, -2)
  line L10 (200.6, -24.3525) -> (200.6, -47.9525) projected
  line L11 (200.6, -29.4975) -> (315.5025, -29.4975)
  line L12 (315.5025, -29.4975) -> (315.5025, -47.5025)
  line L13 (315.5025, -47.5025) -> (296.7525, -47.5025)
  line L14 (296.7525, -47.5025) -> (296.7525, -105.8975)
  line L15 (296.7525, -105.8975) -> (315.5025, -105.8975)
  line L16 (315.5025, -105.8975) -> (315.5025, -123)
  line L17 (216.4009, -123) -> (316, -123) projected
  line L18 (315.5025, -123) -> (216.4009, -123)
  line L19 (216.3009, -120.0025) -> (216.3009, -103.805) projected
  line L20 (216.3009, -103.805) -> (205.25, -103.805) projected
  line L21 (205.25, -103.805) -> (205.25, -86.2525) projected
  line L22 (205.25, -86.2525) -> (215, -86.2525) projected
  line L23 (215, -86.2525) -> (215, -67.1525) projected
  line L24 (215, -67.1525) -> (210.25, -67.1525) projected
  line L25 (210.25, -67.1525) -> (210.25, -48.0525) projected
  line L26 (210.25, -48.0525) -> (200.5, -48.0525) projected
  line L27 (200.5, -48.0525) -> (200.6, -29.4975)
  line L28 (210.1, -2) -> (210.1, -24.3525) projected
  line L29 (210.1, -24.3525) -> (200.6, -24.3525) projected
  line L30 (200.6, -24.3525) -> (200.6, -47.9525) projected
  line L31 (200.6, -47.9525) -> (210.35, -47.9525) projected
  line L32 (210.35, -47.9525) -> (210.35, -67.0525) projected
  line L33 (210.35, -67.0525) -> (215.1, -67.0525) projected
  line L34 (215.1, -67.0525) -> (215.1, -86.3525) projected
  line L35 (215.1, -86.3525) -> (205.35, -86.3525) projected
  line L36 (205.35, -86.3525) -> (205.35, -103.705) projected
  line L37 (205.35, -103.705) -> (216.4009, -103.705) projected
  line L38 (216.4009, -103.705) -> (216.4009, -123) projected
  line L39 (216.4009, -123) -> (316, -123) projected
  line L40 (316, -123) -> (316, -105.8975) projected
  line L41 (316, -2) -> (210.1, -2) projected
  line L42 (277.2225, -76.175) -> (289.7225, -76.175) projected
  line L43 (289.7225, -76.175) -> (289.7225, -82.175) projected
  line L44 (289.7225, -82.175) -> (277.2225, -82.175) projected
  line L45 (277.2225, -82.175) -> (277.2225, -76.175) projected
  line L46 (277.2225, -58.375) -> (277.2225, -52.375) projected
  line L47 (277.2225, -52.375) -> (289.7225, -52.375) projected
  line L48 (289.7225, -52.375) -> (289.7225, -58.375) projected
  line L49 (289.7225, -58.375) -> (277.2225, -58.375) projected
  line L50 (276.9725, -60.2725) -> (290.9775, -60.2725) projected
  line L51 (290.9775, -60.2725) -> (290.9775, -74.2775) projected
  line L52 (290.9775, -74.2775) -> (276.9725, -74.2775) projected
  line L53 (276.9725, -74.2775) -> (276.9725, -60.2725) projected
  line L54 (298.2475, -107.8975) -> (312.2525, -107.8975) projected
  line L55 (312.2525, -107.8975) -> (312.2525, -121.9025) projected
  line L56 (312.2525, -121.9025) -> (298.2475, -121.9025) projected
  line L57 (298.2475, -121.9025) -> (298.2475, -107.8975) projected
  line L58 (279.2475, -107.8975) -> (293.2525, -107.8975) projected
  line L59 (293.2525, -107.8975) -> (293.2525, -121.9025) projected
  line L60 (293.2525, -121.9025) -> (279.2475, -121.9025) projected
  line L61 (279.2475, -121.9025) -> (279.2475, -107.8975) projected
  line L62 (260.2475, -107.8975) -> (274.2525, -107.8975) projected
  line L63 (274.2525, -107.8975) -> (274.2525, -121.9025) projected
  line L64 (274.2525, -121.9025) -> (260.2475, -121.9025) projected
  line L65 (260.2475, -121.9025) -> (260.2475, -107.8975) projected
  line L66 (241.2475, -107.8975) -> (255.2525, -107.8975) projected
  line L67 (255.2525, -107.8975) -> (255.2525, -121.9025) projected
  line L68 (255.2525, -121.9025) -> (241.2475, -121.9025) projected
  line L69 (241.2475, -121.9025) -> (241.2475, -107.8975) projected
  line L70 (219.2475, -107.8975) -> (233.2525, -107.8975) projected
  line L71 (233.2525, -107.8975) -> (233.2525, -121.9025) projected
  line L72 (233.2525, -121.9025) -> (219.2475, -121.9025) projected
  line L73 (219.2475, -121.9025) -> (219.2475, -107.8975) projected
  line L74 (279.2475, -88.7975) -> (293.2525, -88.7975) projected
  line L75 (293.2525, -88.7975) -> (293.2525, -102.8025) projected
  line L76 (293.2525, -102.8025) -> (279.2475, -102.8025) projected
  line L77 (279.2475, -102.8025) -> (279.2475, -88.7975) projected
  line L78 (252.9975, -88.7975) -> (267.0025, -88.7975) projected
  line L79 (267.0025, -88.7975) -> (267.0025, -102.8025) projected
  line L80 (267.0025, -102.8025) -> (252.9975, -102.8025) projected
  line L81 (252.9975, -102.8025) -> (252.9975, -88.7975) projected
  line L82 (226.7475, -88.7975) -> (240.7525, -88.7975) projected
  line L83 (240.7525, -88.7975) -> (240.7525, -102.8025) projected
  line L84 (240.7525, -102.8025) -> (226.7475, -102.8025) projected
  line L85 (226.7475, -102.8025) -> (226.7475, -88.7975) projected
  line L86 (207.7475, -88.7975) -> (221.7525, -88.7975) projected
  line L87 (221.7525, -88.7975) -> (221.7525, -102.8025) projected
  line L88 (221.7525, -102.8025) -> (207.7475, -102.8025) projected
  line L89 (207.7475, -102.8025) -> (207.7475, -88.7975) projected
  line L90 (255.4975, -69.6975) -> (269.5025, -69.6975) projected
  line L91 (269.5025, -69.6975) -> (269.5025, -83.7025) projected
  line L92 (269.5025, -83.7025) -> (255.4975, -83.7025) projected
  line L93 (255.4975, -83.7025) -> (255.4975, -69.6975) projected
  line L94 (236.4975, -69.6975) -> (250.5025, -69.6975) projected
  line L95 (250.5025, -69.6975) -> (250.5025, -83.7025) projected
  line L96 (250.5025, -83.7025) -> (236.4975, -83.7025) projected
  line L97 (236.4975, -83.7025) -> (236.4975, -69.6975) projected
  line L98 (217.4975, -69.6975) -> (231.5025, -69.6975) projected
  line L99 (231.5025, -69.6975) -> (231.5025, -83.7025) projected
  line L100 (231.5025, -83.7025) -> (217.4975, -83.7025) projected
  line L101 (217.4975, -83.7025) -> (217.4975, -69.6975) projected
  line L102 (250.7475, -50.7441) -> (264.7525, -50.7441) projected
  line L103 (264.7525, -50.7441) -> (264.7525, -64.7491) projected
  line L104 (264.7525, -64.7491) -> (250.7475, -64.7491) projected
  line L105 (250.7475, -64.7491) -> (250.7475, -50.7441) projected
  line L106 (231.7475, -50.7475) -> (245.7525, -50.7475) projected
  line L107 (245.7525, -50.7475) -> (245.7525, -64.7525) projected
  line L108 (245.7525, -64.7525) -> (231.7475, -64.7525) projected
  line L109 (231.7475, -64.7525) -> (231.7475, -50.7475) projected
  line L110 (212.7475, -50.5975) -> (226.7525, -50.5975) projected
  line L111 (226.7525, -50.5975) -> (226.7525, -64.6025) projected
  line L112 (226.7525, -64.6025) -> (212.7475, -64.6025) projected
  line L113 (212.7475, -64.6025) -> (212.7475, -50.5975) projected
  line L114 (297.9975, -31.4975) -> (312.0025, -31.4975) projected
  line L115 (312.0025, -31.4975) -> (312.0025, -45.5025) projected
  line L116 (312.0025, -45.5025) -> (297.9975, -45.5025) projected
  line L117 (297.9975, -45.5025) -> (297.9975, -31.4975) projected
  line L118 (278.9975, -31.4975) -> (293.0025, -31.4975) projected
  line L119 (293.0025, -31.4975) -> (293.0025, -45.5025) projected
  line L120 (293.0025, -45.5025) -> (278.9975, -45.5025) projected
  line L121 (278.9975, -45.5025) -> (278.9975, -31.4975) projected
  line L122 (259.9975, -31.4975) -> (274.0025, -31.4975) projected
  line L123 (274.0025, -31.4975) -> (274.0025, -45.5025) projected
  line L124 (274.0025, -45.5025) -> (259.9975, -45.5025) projected
  line L125 (259.9975, -45.5025) -> (259.9975, -31.4975) projected
  line L126 (240.9975, -31.4975) -> (255.0025, -31.4975) projected
  line L127 (255.0025, -31.4975) -> (255.0025, -45.5025) projected
  line L128 (255.0025, -45.5025) -> (240.9975, -45.5025) projected
  line L129 (240.9975, -45.5025) -> (240.9975, -31.4975) projected
  line L130 (221.9975, -31.4975) -> (236.0025, -31.4975) projected
  line L131 (236.0025, -31.4975) -> (236.0025, -45.5025) projected
  line L132 (236.0025, -45.5025) -> (221.9975, -45.5025) projected
  line L133 (221.9975, -45.5025) -> (221.9975, -31.4975) projected
  line L134 (202.9975, -31.4975) -> (217.0025, -31.4975) projected
  line L135 (217.0025, -31.4975) -> (217.0025, -45.5025) projected
  line L136 (217.0025, -45.5025) -> (202.9975, -45.5025) projected
  line L137 (202.9975, -45.5025) -> (202.9975, -31.4975) projected
  line L138 (296.4975, -2.9975) -> (310.5025, -2.9975) projected
  line L139 (310.5025, -2.9975) -> (310.5025, -17.0025) projected
  line L140 (310.5025, -17.0025) -> (296.4975, -17.0025) projected
  line L141 (296.4975, -17.0025) -> (296.4975, -2.9975) projected
  line L142 (262.9975, -2.9975) -> (277.0025, -2.9975) projected
  line L143 (277.0025, -2.9975) -> (277.0025, -17.0025) projected
  line L144 (277.0025, -17.0025) -> (262.9975, -17.0025) projected
  line L145 (262.9975, -17.0025) -> (262.9975, -2.9975) projected
  line L146 (238.9975, -2.9975) -> (253.0025, -2.9975) projected
  line L147 (253.0025, -2.9975) -> (253.0025, -17.0025) projected
  line L148 (253.0025, -17.0025) -> (238.9975, -17.0025) projected
  line L149 (238.9975, -17.0025) -> (238.9975, -2.9975) projected
  line L150 (214.9975, -2.9975) -> (229.0025, -2.9975) projected
  line L151 (229.0025, -2.9975) -> (229.0025, -17.0025) projected
  line L152 (229.0025, -17.0025) -> (214.9975, -17.0025) projected
  line L153 (214.9975, -17.0025) -> (214.9975, -2.9975) projected
  line L154 (316, -105.8975) -> (296.7525, -105.8975) projected
  line L155 (296.7525, -105.8975) -> (296.7525, -47.5025) projected
  line L156 (296.7525, -47.5025) -> (316, -47.5025) projected
  line L157 (316, -47.5025) -> (316, -2) projected
  line L158 (296.7525, -105.8975) -> (296.7525, -47.5025) projected
  line L159 (278.0025, -2) -> (278.0025, -5)
  line L160 (278.0025, -5) -> (280.5025, -5)
  line L161 (280.5025, -5) -> (280.5025, -19.0025)
  point P0 (0, 0)
  point P1 (314.0025, -2)
  dimension "d63" = 2
  dimension "d64" = 2
  dimension "d65" = 3.5
  dimension "d66" = 3.5
  dimension "d67" = 3.5
  dimension "d68" = 3.5
  dimension "d69" = 2
  dimension "d71" = 2
  dimension "d94" = 3
  dimension "d95" = 1
  constraints: 38 end point, 11 perpendicular, 11 point on line, 4 collinear, 1 horizontal, 1 parallel
  measures "d63" distance between parallel lines of L1 L152
  measures "d64" distance between parallel lines of L134 L11
  measures "d65" distance between parallel lines of L2 L143
  measures "d66" distance between parallel lines of L141 L6
  measures "d67" distance between parallel lines of L8 L139
  measures "d68" distance between parallel lines of L12 L115
  measures "d69" distance between parallel lines of L13 L116
  measures "d71" distance between parallel lines of L15 L54
  measures "d94" distance between parallel lines of L160 L3
  measures "d95" distance between parallel lines of L159 L143
extrude "Extrusion2" add sketch "Sketch2" along normal blind 2.5 contours L3 L159 L160 L161 L1 L0 | L5 L8 L7 L6 | L11 L12 L13 L14 L15 L16 L17 L38 L37 L36 L35 L34 L33 L32 L31 L10
sketch "Sketch3" plane through (0, 0, 0) normal (0, 0, -1) x (-1, 0, 0)
  line L0 (-277.2225, -52.375) -> (-289.7225, -52.375) construction
  line L1 (-277.2225, -58.375) -> (-277.2225, -52.375) construction
  line L2 (-289.7225, -52.375) -> (-289.7225, -58.375) construction
  line L3 (-289.7225, -58.375) -> (-277.2225, -58.375) construction
  line L4 (-289.7225, -76.175) -> (-289.7225, -82.175) construction
  line L5 (-277.2225, -76.175) -> (-289.7225, -76.175) construction
  line L6 (-277.2225, -82.175) -> (-277.2225, -76.175) construction
  line L7 (-289.7225, -82.175) -> (-277.2225, -82.175) construction
  line L8 (-291.7225, -52.375) -> (-274.2225, -52.375)
  line L9 (-274.2225, -52.375) -> (-274.2225, -82.175)
  line L10 (-274.2225, -82.175) -> (-291.7225, -82.175)
  line L11 (-291.7225, -82.175) -> (-291.7225, -76.175)
  line L12 (-291.7225, -76.175) -> (-280.9725, -76.175)
  line L13 (-280.9725, -76.175) -> (-280.9725, -58.375)
  line L14 (-280.9725, -58.375) -> (-291.7225, -58.375)
  line L15 (-291.7225, -52.375) -> (-291.7225, -58.375)
  line L16 (-276.9725, -74.2775) -> (-276.9725, -60.2725) projected
  point P0 (0, 0)
  dimension "d74" = 4
  dimension "d75" = 3
  dimension "d76" = 2
  constraints: 16 end point, 6 point on line, 4 perpendicular, 1 collinear
  measures "d74" distance between parallel lines of L16 L13
  measures "d75" distance between parallel lines of L9 L1
  measures "d76" distance between parallel lines of L15 L2
extrude "Extrusion3" cut sketch "Sketch3" against normal blind 2
sketch "Sketch4" plane through (0, 0, 3) normal (0, 0, 1) x (1, 0, 0)
  line L0 (277.2225, -58.375) -> (277.2225, -52.375) construction
  line L1 (277.2225, -82.175) -> (277.2225, -76.175) construction
  line L2 (277.2225, -56.375) -> (276.2225, -56.375)
  line L3 (276.2225, -56.375) -> (276.2225, -54.375)
  line L4 (276.2225, -54.375) -> (277.2225, -54.375)
  line L5 (277.2225, -54.375) -> (277.2225, -56.375)
  line L6 (277.2225, -80.175) -> (276.2225, -80.175)
  line L7 (276.2225, -80.175) -> (276.2225, -78.175)
  line L8 (276.2225, -78.175) -> (277.2225, -78.175)
  line L9 (277.2225, -78.175) -> (277.2225, -80.175)
  point P0 (0, 0)
  point P1 (277.2225, -55.375)
  point P2 (277.2225, -79.175)
  dimension "d83" = 1
  dimension "d84" = 2
  dimension "d85" = 1
  dimension "d86" = 2
  constraints: 16 end point, 4 midpoint, 4 parallel, 2 horizontal, 2 perpendicular, 2 point on line
  measures "d83" distance of L3.end L4.end
  measures "d84" distance of L2.end L3.end
  measures "d85" distance of L7.end L8.end
  measures "d86" distance of L6.end L7.end
extrude "Extrusion4" cut sketch "Sketch4" against normal up to surface (3 mm away)
sketch "Sketch7" plane through (0, 0, 3) normal (0, 0, 1) x (1, 0, 0)
  line L0 (216.4009, -123) -> (218.4009, -123)
  line L1 (218.4009, -123) -> (218.4009, -120)
  line L2 (218.4009, -120) -> (216.4009, -120)
  line L3 (216.4009, -120) -> (216.4009, -123)
  line L4 (278.2475, -125.1025) -> (278.2475, -120.0525) construction
  line L5 (278.2475, -120.0525) -> (275.2475, -120.0525)
  line L6 (275.2475, -120.0525) -> (275.2475, -117.0525)
  line L7 (275.2475, -117.0525) -> (278.2475, -117.0525)
  line L8 (278.2475, -117.0525) -> (278.2475, -120.0525)
  point P0 (0, 0)
  dimension "d96" = 2
  dimension "d97" = 3
  dimension "d98" = 3
  dimension "d99" = 3
  constraints: 16 end point, 4 parallel, 2 horizontal, 2 perpendicular
  measures "d96" distance of L1.end L2.end
  measures "d97" distance of L0.end L1.end
  measures "d98" distance of L6.end L7.end
  measures "d99" distance of L5.end L6.end
extrude "Extrusion7" cut sketch "Sketch7" against normal blind 2
equation "\"d1\" = d0"
equation "\"d2\" = sw"
equation "\"d3\" = sw"
equation "\"d4\" = sw"
equation "\"d5\" = sw"
equation "\"d6\" = sw"
equation "\"d7\" = sw"
equation "\"d8\" = sw"
equation "\"d9\" = sw"
equation "\"d10\" = sw"
equation "\"d11\" = sw"
equation "\"d12\" = sw"
equation "\"d13\" = sw"
equation "\"d14\" = sw"
equation "\"d15\" = sw"
equation "\"d16\" = sw"